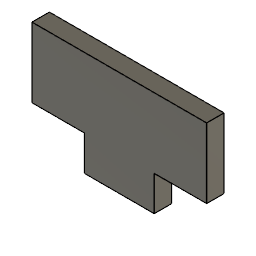
vertical divider (Autodesk Fusion 360 design; units mm, degrees)
Autodesk Fusion 360 part; units mm, degrees
sketch "Sketch1" plane through (0, 0, 0) normal (0, 1, 0) x (-1, 0, 0)
  line L0 (-5, 0) -> (5, 0)
  line L1 (5, 0) -> (5, 5)
  line L2 (5, 5) -> (12.5, 5)
  line L3 (12.5, 5) -> (12.5, 15)
  line L4 (12.5, 15) -> (-12.5, 15)
  line L5 (-12.5, 15) -> (-12.5, 5)
  line L6 (-12.5, 5) -> (-5, 5)
  line L7 (-5, 5) -> (-5, 0)
  point P0 (0, 15)
  dimension "d2" = 25
  dimension "d3" = 10
  dimension "d4" = 5
  dimension "d5" = 10
  constraint horizontal L0
  constraint perpendicular L0 L1
  constraint perpendicular L1 L2
  constraint perpendicular L2 L3
  constraint perpendicular L3 L4
  constraint perpendicular L4 L5
  constraint perpendicular L5 L6
  constraint perpendicular L6 L7
  constraint coincident L1.end L6
  constraint midpoint L4 P0
  constraint midpoint L0 origin
  constraint vertical P0 origin
  measures "d2" distance of L3.end L4.end
  measures "d3" distance of L0.end L0.start
  measures "d4" distance of L0.end L1.end
  measures "d5" distance of L2.end L3.end
extrude "Extrude1" add sketch "Sketch1" along normal mid plane 2.5
